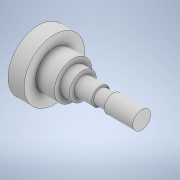
# Autodesk Inventor part: Sketch 2d terminado sin rotacion aun
Saved by Autodesk Inventor 2021 (Build 250183000, 183)
## iProperties
Created: 2020-12-31
Part Number: Sketch 2d terminado sin rotacion aun
Material: Generic
Document SubType Name: Modeling
Designer: dieku
Density: 1 g/cm^3
Appearance: Default
Author: dieku
Autodesk Inventor part; units mm, degrees
ref_plane "YZ Plane" through (0, 0, 0) normal (1, 0, 0) x (0, 1, 0)
ref_plane "XZ Plane" through (0, 0, 0) normal (0, 1, 0) x (-1, 0, 0)
ref_plane "XY Plane" through (0, 0, 0) normal (0, 0, 1) x (1, 0, 0)
sketch "Sketch1" plane through (0, 0, 0) normal (0, 0, 1) x (1, 0, 0)
  line L0 (60, 13.5) -> (60, 0) construction
  line L1 (60, 0) -> (60, 34)
  line L2 (60, 34) -> (78, 34)
  line L3 (78, 34) -> (78, 0)
  line L4 (78, 0) -> (78, 21)
  line L5 (78, 21) -> (99, 21)
  line L6 (99, 21) -> (99, 0)
  line L7 (99, 0) -> (99, 15)
  line L8 (99, 15) -> (110, 15)
  line L9 (110, 15) -> (110, 0)
  line L10 (110, 0) -> (110, 10)
  line L11 (110, 10) -> (130, 10)
  line L12 (130, 10) -> (130, 0)
  line L13 (130, 0) -> (130, 8)
  line L14 (130, 8) -> (144, 8)
  line L15 (144, 8) -> (144, 0)
  line L16 (144, 0) -> (144, 10)
  line L17 (144, 10) -> (176, 10)
  line L18 (176, 10) -> (176, 0)
  line L19 (0, 0) -> (225.6875, 0)
  dimension "d8" = 34
  dimension "d9" = 18
  dimension "d10" = 21
  dimension "d11" = 21
  dimension "d12" = 15
  dimension "d13" = 11
  dimension "d14" = 10
  dimension "d15" = 20
  dimension "d16" = 8
  dimension "d17" = 14
  dimension "d18" = 10
  dimension "d19" = 32
  dimension "d46" = 98
  constraints: 40 end point, 12 perpendicular, 5 point on line, 2 vertical, 1 horizontal
  measures "d8" distance of L0.end L1.end
  measures "d9" distance of L1.end L2.end
  measures "d10" distance of L3.end L4.end
  measures "d11" distance of L4.end L5.end
  measures "d12" distance of L6.end L7.end
  measures "d13" distance of L7.end L8.end
  measures "d14" distance of L9.end L10.end
  measures "d15" distance of L10.end L11.end
  measures "d16" distance of L12.end L13.end
  measures "d17" distance of L13.end L14.end
  measures "d18" distance of L15.end L16.end
  measures "d19" distance of L16.end L17.end
  measures "d46" horizontal distance of L17.end L2.end
revolve "Revolution1" add sketch "Sketch1" angle 360 about axis through (0, 0, 0) along (1, 0, 0)
sketch "Sketch4" plane through (60, 0, 0) normal (-1, 0, 0) x (0, 0, 1)
  point P0 (0, 0)
body "Solid1"
